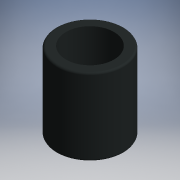
# Autodesk Inventor part: 242770 EAGF 25x35x40---(B)
Saved by Autodesk Inventor 2017.3 (Build 213256000, 256)
## iProperties
Part Number: 242770 EAGF 25x35x40---(B)
Material: Generic
Catalog Web Link: www.cadenas.de
Description: EAGF-(B)-Kugelbuchse
Vendor: FESTO
Document SubType Name: Modeling
Designer: partserver
Manufacturer: FESTO
Mass: 18.803 g
Surface Area: 83.8702 cm^2
Volume: 18.803 cm^3
Density: 1 g/cm^3
Appearance: PSOLRGB-45-51-51
Category: PARTsolutions
Company: FESTO
Title: 242770 EAGF 25x35x40---(B)
Author: Cadenas PARTsolutions
Comments: Kugelbuchse
PSOL_IDENT_0: {$CADENAS_DATA\23d-libs\festo\parts\e\eagf\parts\eagf_kubu.prj},194 {VTYP=3D},{NB=242770 EAGF 25x35x
PSOL_IDENT_1: 40---(B)},{LINA=242770 EAGF 25x35x40---(B)},{NN=EAGF-(B)},{DATE=20.07.2020 13:53:58},{GEOMDATE=02.09
PSOL_IDENT_2: .2015 14:27:16},{VERSION=},{LINEID=20},{WBVAR=},{WBNUMERIC=}  {NB=242770 EAGF 25x35x40---(B)},{LINA=
PSOL_IDENT_3: 242770 EAGF 25x35x40---(B)},{KT=DUMMY},{TNR=242770},{TYP=EAGF 25x35x40},{D1=35.000},{D2=25.000},{L=4
PSOL_IDENT_4: 0.000}
NB: 242770 EAGF 25x35x40---(B)
NN: EAGF-(B)
NT: Kugelbuchse
NBSYN: $TNR. $TYP.---(B)
LINA: 242770 EAGF 25x35x40---(B)
CATALOG: Festo
TNR: 242770
TYP: EAGF 25x35x40
D1: 35
D2: 25
L: 40
SUPPLIER: FESTO
ARTICLENO: 242770 EAGF 25x35x40---(B)
BOMINFO: 242770 EAGF 25x35x40---(B)
CREATOR: CADENAS GmbH
Autodesk Inventor part; units mm, degrees
sketch "Sketch_1" plane through (0, 0, 0) normal (1, 0, 0) x (0, 1, 0)
  line L0 (0, -40) -> (0, 0)
  line L1 (12.5, 0) -> (12.5, -40)
  line L2 (12.5, -40) -> (16.5, -40)
  arc A0 (16.5, -40) -> (17.5, -39) centre (16.5, -39) ccw
  line L3 (17.5, -39) -> (17.5, -1)
  arc A1 (17.5, -1) -> (16.5, 0) centre (16.5, -1) ccw
  line L4 (16.5, 0) -> (12.5, 0)
  constraints: 10 end point, 4 point on circle, 2 centre point
revolve "Revolution1" add sketch "Sketch_1" angle 360 about axis through (0, 0, -40) along (0, 0, -1)
ref_plane "ANBAU_XY" through (0, 0, 0) normal (0, 0, -1) x (1, 0, 0)
ref_plane "ANBAU_YZ" through (0, 0, 0) normal (1, 0, 0) x (0, -1, 0)
ref_plane "ANBAU_ZX" through (0, 0, 0) normal (0, -1, 0) x (0, 0, -1)
body "Solid1"
